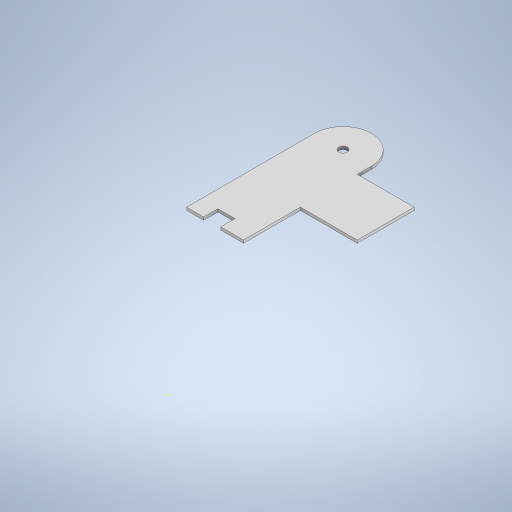
# Autodesk Inventor part: Otomasi Part2
Saved by Autodesk Inventor 2023 (Build 270158000, 158)
## iProperties
Created: 2024-05-22
Part Number: Otomasi Part2
Material: Generic
Document SubType Name: Modeling
Designer: ASUS
Density: 1 g/cm^3
Appearance: Default
Author: ASUS
Autodesk Inventor part; units mm, degrees
ref_plane "YZ Plane" through (0, 0, 0) normal (1, 0, 0) x (0, 1, 0)
ref_plane "XZ Plane" through (0, 0, 0) normal (0, 1, 0) x (-1, 0, 0)
ref_plane "XY Plane" through (0, 0, 0) normal (0, 0, 1) x (1, 0, 0)
sketch "Sketch1" plane through (0, 0, 0) normal (0, 0, 1) x (1, 0, 0)
  point P0 (0, 0)
sketch "Sketch2" plane through (0, 0, 0) normal (0, 0, 1) x (1, 0, 0)
  point P0 (0, 0)
sketch "Sketch3" plane through (0, 0, 0) normal (0, 1, 0) x (-1, 0, 0)
  line L0 (265.7025, -96.8628) -> (235.7025, -96.8628)
  line L1 (235.7025, -96.8628) -> (235.7025, -121.8628)
  line L2 (235.7025, -121.8628) -> (205.7025, -121.8628)
  line L3 (205.7025, -121.8628) -> (205.7025, -96.8628)
  line L4 (205.7025, -96.8628) -> (165.7025, -96.8628)
  line L5 (165.7025, -96.8628) -> (65.7025, -96.8628)
  line L6 (65.7025, -96.8628) -> (65.7025, -196.8628)
  line L7 (65.7025, -196.8628) -> (165.7025, -196.8628)
  line L8 (165.7025, -196.8628) -> (165.7025, -396.8628)
  line L9 (165.7025, -396.8628) -> (65.7025, -396.8628)
  line L10 (65.7025, -396.8628) -> (65.7025, -496.8628)
  line L11 (65.7025, -496.8628) -> (165.7025, -496.8628)
  line L12 (165.7025, -496.8628) -> (165.7025, -521.8628)
  line L13 (265.7025, -96.8628) -> (265.7025, -521.8628)
  arc A0 (165.7025, -521.8628) -> (265.7025, -521.8628) centre (215.7025, -521.8628) ccw
  circle A1 centre (215.7025, -521.8628) radius 7.5
  point P0 (0, 0)
  dimension "d0" = 30
  dimension "d1" = 25
  dimension "d2" = 30
  dimension "d3" = 40
  dimension "d4" = 100
  dimension "d5" = 100
  dimension "d6" = 200
  dimension "d7" = 100
  dimension "d8" = 25
  dimension "d9" = 15
  constraints: 28 end point, 7 perpendicular, 7 point on line, 2 centre point, 2 point on circle, 2 tangent, 2 vertical, 1 coincident, 1 horizontal
  measures "d0" distance of L0.start L0.end
  measures "d1" distance of L0.end L1.end
  measures "d2" distance of L1.end L2.end
  measures "d3" distance of L3.end L4.end
  measures "d4" distance of L4.end L5.end
  measures "d5" distance of L5.end L6.end
  measures "d6" distance of L7.end L8.end
  measures "d7" distance of L9.end L10.end
  measures "d8" distance of L11.end L12.end
  measures "d9" diameter of A1
extrude "Extrusion1" add sketch "Sketch3" along normal blind 5
sketch "Sketch4" plane through (0, 5, 0) normal (0, 1, 0) x (1, 0, 0)
  line L0 (-165.7025, 196.8628) -> (-165.7025, 296.8628)
  line L1 (-165.7025, 196.8628) -> (-165.7025, 396.8628) projected
  line L2 (-265.7025, 521.8628) -> (-265.7025, 96.8628) projected
  line L3 (-265.7025, 296.8628) -> (-235.7025, 296.8628)
  line L4 (-235.7025, 296.8628) -> (-235.7025, 321.8628)
  line L5 (-235.7025, 321.8628) -> (-205.7025, 321.8628)
  line L6 (-205.7025, 321.8628) -> (-205.7025, 296.8628)
  line L7 (-265.7025, 96.8628) -> (-265.7025, 296.8628)
  line L8 (-235.7025, 96.8628) -> (-235.7025, 121.8628) projected
  line L9 (-265.7025, 96.8628) -> (-235.7025, 96.8628)
  line L10 (-235.7025, 96.8628) -> (-235.7025, 121.8628)
  line L11 (-235.7025, 121.8628) -> (-205.7025, 121.8628)
  line L12 (-205.7025, 121.8628) -> (-205.7025, 96.8628)
  line L13 (-205.7025, 96.8628) -> (-65.7025, 96.8628) projected
  line L14 (-205.7025, 96.8628) -> (-65.7025, 96.8628)
  line L15 (-65.7025, 96.8628) -> (-65.7025, 196.8628) projected
  line L16 (-65.7025, 96.8628) -> (-65.7025, 196.8628)
  line L17 (-65.7025, 196.8628) -> (-165.7025, 196.8628) projected
  line L18 (-65.7025, 196.8628) -> (-165.7025, 196.8628)
  line L19 (-165.7025, 296.8628) -> (-205.7025, 296.8628)
  line L20 (-235.7025, 296.8628) -> (-265.7025, 296.8628)
  point P0 (0, 0)
  dimension "d12" = 100
  dimension "d13" = 30
  dimension "d15" = 30
  constraints: 30 end point, 9 perpendicular, 4 collinear, 2 point on line, 1 horizontal, 1 midpoint
  measures "d12" distance of L0.start L0.end
  measures "d13" distance of L3.start L3.end
  measures "d15" distance of L4.end L5.end
extrude "Extrusion2" cut sketch "Sketch4" against normal blind 10
body "Solid1"
